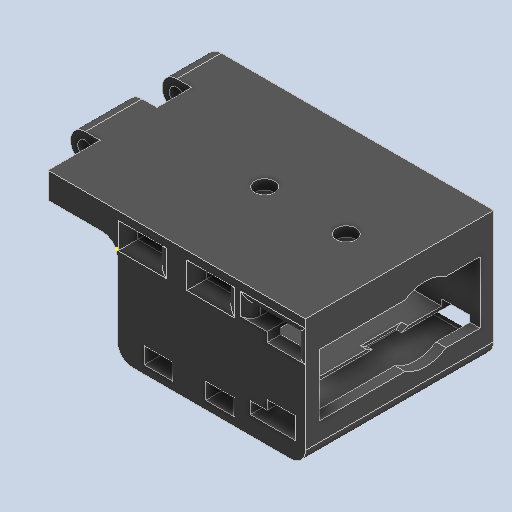
# Autodesk Inventor part: Base - version 2
Saved by Autodesk Inventor 2026 (Build 300175050, 175E)
## iProperties
Created: 2025-10-13
Part Number: Base - version 2
Material: Plastico PETG
Document SubType Name: Modeling
Designer: bello
Density: 1.27 g/cm^3
Appearance: Genérico
Author: bello
Autodesk Inventor part; units mm, degrees
ref_plane "YZ Plane" through (0, 0, 0) normal (1, 0, 0) x (0, 1, 0)
sketch "Boceto1" plane through (0, 0, 0) normal (0, 1, 0) x (-1, 0, 0)
  line L0 (0, 0) -> (-38, 0)
  line L1 (-38, 0) -> (-38, -38)
  line L2 (-38, -38) -> (0, -38)
  line L3 (0, -38) -> (0, 0)
  dimension "d0" = 38
  dimension "d1" = 38
  constraints: 8 end point, 2 parallel, 1 horizontal, 1 perpendicular
  measures "d0" distance of L2.end L0.start
  measures "d1" distance of L0.start L0.end
extrude "Extrusión1" add sketch "Boceto1" along normal blind 26
sketch "Boceto2" plane through (38, 0, 0) normal (1, 0, 0) x (0, 0, -1)
  line L0 (7.25, 19.25) -> (30.75, 19.25)
  line L1 (30.75, 19.25) -> (30.75, 6.75)
  line L2 (30.75, 6.75) -> (7.25, 6.75)
  line L3 (7.25, 6.75) -> (7.25, 19.25)
  line L4 (0, 26) -> (38, 26) projected
  line L5 (19, 26) -> (19, 0)
  line L6 (0, 0) -> (38, 0) projected
  line L7 (0, 0) -> (0, 26) projected
  line L8 (0, 13) -> (38, 13)
  line L9 (38, 0) -> (38, 26) projected
  dimension "d4" = 23.5
  dimension "d5" = 12.5
  dimension "d6" = 23.5
  dimension "d7" = 12.5
  constraints: 12 end point, 4 midpoint, 2 parallel, 1 horizontal, 1 perpendicular
  measures "d4" distance of L0.start L0.end
  measures "d5" distance of L2.end L0.start
  measures "d6" diameter of L3 L5
  measures "d7" diameter of L2 L8
extrude "Extrusión2" cut sketch "Boceto2" against normal blind 36.5 contours L0 L5 L8 L3 | L0 L1 L8 L5 | L8 L5 L2 L3 | L8 L1 L2 L5
sketch "Boceto3" plane through (38, 0, 0) normal (1, 0, 0) x (0, 0, -1)
  line L0 (7.25, 19.25) -> (30.75, 19.25) projected
  line L1 (19, 19.25) -> (19, 6.75)
  line L2 (30.75, 6.75) -> (7.25, 6.75) projected
  line L3 (2.75, 6.75) -> (35.25, 6.75)
  line L4 (35.25, 6.75) -> (35.25, 19.25)
  line L5 (35.25, 19.25) -> (2.75, 19.25)
  line L6 (2.75, 19.25) -> (2.75, 6.75)
  line L7 (2.75, 6.75) -> (35.25, 19.25) construction
  line L8 (35.25, 6.75) -> (2.75, 19.25) construction
  point P0 (0, 0)
  point P1 (19, 13)
  point P2 (7.25, 6.75)
  point P3 (7.25, 19.25)
  dimension "d10" = 32.5
  constraints: 14 end point, 5 midpoint, 2 parallel, 1 horizontal, 1 perpendicular
  measures "d10" distance of L5.end L4.end
extrude "Extrusión3" cut sketch "Boceto3" against normal blind 19
sketch "Boceto5" plane through (19, 0, 0) normal (1, 0, 0) x (0, 0, -1)
  line L0 (2.75, 6.75) -> (2.75, 19.25) projected
  line L1 (2.75, 13) -> (35.25, 13)
  line L2 (35.25, 19.25) -> (35.25, 6.75) projected
  line L3 (7.25, 19.25) -> (7.25, 6.75) projected
  circle A0 centre (5.35, 13) radius 0.8
  circle A1 centre (32.65, 13) radius 0.8
  point P0 (0, 0)
  dimension "d16" = 4.5
  dimension "d17" = 1.6
  dimension "d18" = 2.6
  dimension "d19" = 2.6
  dimension "d20" = 1.6
  constraints: 2 centre point, 2 end point, 2 midpoint, 2 point on line
  measures "d16" distance between parallel lines of L3 L0
  measures "d17" diameter of A0
  measures "d18" distance from line of L0 A0.centre
  measures "d19" distance from line of L2 A1.centre
  measures "d20" diameter of A1
extrude "Extrusión5" cut sketch "Boceto5" against normal blind 5.7
sketch "Boceto6" plane through (38, 0, 0) normal (1, 0, 0) x (0, 0, -1)
  line L0 (0, 0) -> (0, 26) projected
  line L1 (0, 13) -> (38, 13)
  line L2 (38, 0) -> (38, 26) projected
  circle A0 centre (24.25, 13) radius 7.5
  line L3 (2.75, 6.75) -> (2.75, 19.25) projected
  line L4 (35.25, 19.25) -> (35.25, 6.75) projected
  dimension "d24" = 15
  dimension "d30" = 11
  constraints: 2 end point, 2 midpoint, 1 centre point, 1 point on line
  measures "d24" diameter of A0
  measures "d30" distance from line of L4 A0.centre
extrude "Extrusión6" cut sketch "Boceto6" against normal blind 9
sketch "Boceto9" plane through (38, 0, 0) normal (1, 0, 0) x (0, 0, -1)
  line L0 (28.9453, 7.1) -> (48.9575, 7.1)
  arc A0 (28.3958, 19.25) -> (20.1042, 19.25) centre (24.25, 13) ccw projected
  circle A1 centre (24.25, 13) radius 3.7369
  line L1 (29.3531, 3.4386) -> (49.9663, 3.4386)
  point P0 (0, 0)
  dimension "d31" = 5.9
  dimension "d32" = 3.6614
  dimension "d33" = 9.0792
  constraints: 4 end point, 2 horizontal, 1 centre point, 1 coincident
  measures "d31" distance from line of L0 A1.centre
  measures "d32" distance between parallel lines of L1 L0
sketch "Boceto12" plane through (38, 0, -38) normal (0, 0, -1) x (-1, 0, 0)
  line L0 (31.8255, 18) -> (36.5, 18)
  line L1 (36.5, 18) -> (36.5, 8)
  line L2 (36.5, 8) -> (31.8255, 8)
  line L3 (31.8255, 8) -> (31.8255, 18)
  line L4 (38, 0) -> (38, 26) projected
  line L5 (38, 13) -> (26.3791, 13)
  dimension "d52" = 1.5
  dimension "d57" = 5
  dimension "d58" = 10
  constraints: 10 end point, 2 horizontal, 2 parallel, 1 midpoint, 1 perpendicular
  measures "d52" distance between parallel lines of L1 L4
  measures "d57" distance between parallel lines of L5 L0
  measures "d58" distance of L2.end L0.start
extrude "Extrusión10" cut sketch "Boceto12" against normal blind 10
sketch "Boceto10" plane through (38, 0, -38) normal (0, 0, -1) x (-1, 0, 0)
  line L0 (2.05, 8) -> (7.75, 8)
  line L1 (7.75, 8) -> (7.75, 3.7)
  line L2 (7.75, 3.7) -> (2.05, 3.7)
  line L3 (2.05, 3.7) -> (2.05, 8)
  line L4 (0, 0) -> (0, 26) projected
  line L5 (38, 0) -> (38, 26) projected
  line L6 (0, 0) -> (38, 0) projected
  line L7 (14.45, 1.7) -> (20.15, 1.7)
  line L8 (20.15, 1.7) -> (20.15, 5)
  line L9 (20.15, 5) -> (14.45, 5)
  line L10 (14.45, 5) -> (14.45, 1.7)
  line L11 (26.85, 1.7) -> (32.55, 1.7)
  line L12 (32.55, 1.7) -> (32.55, 5)
  line L13 (32.55, 5) -> (26.85, 5)
  line L14 (26.85, 5) -> (26.85, 1.7)
  line L15 (38, 13) -> (0, 13)
  line L16 (7.75, 3.7) -> (11.15, 3.7)
  line L17 (11.15, 3.7) -> (11.15, 6.1)
  line L18 (11.15, 6.1) -> (7.75, 6.1)
  line L19 (7.75, 6.1) -> (7.75, 3.7)
  line L20 (2.05, 8) -> (7.75, 3.7)
  line L21 (7.75, 8) -> (2.05, 3.7)
  line L22 (14.45, 5) -> (20.15, 1.7)
  line L23 (14.45, 1.7) -> (20.15, 5)
  line L24 (26.85, 5) -> (32.55, 1.7)
  line L25 (26.85, 1.7) -> (32.55, 5)
  point P0 (29.7, 3.35)
  point P1 (17.3, 3.35)
  point P2 (4.9, 5.85)
  dimension "d35" = 4.3
  dimension "d36" = 5.7
  dimension "d39" = 2.05
  dimension "d49" = 3.3
  dimension "d59" = 5
  dimension "d61" = 3.7
  dimension "d62" = 1.7
  dimension "d63" = 6.7
  dimension "d64" = 6.7
  dimension "d65" = 5.7
  dimension "d66" = 5.7
  dimension "d67" = 3.3
  dimension "d134" = 3.4
  dimension "d135" = 2.4
  dimension "d148" = 8.3
  dimension "d149" = 20.7
  dimension "d150" = 4.9
  constraints: 46 end point, 8 parallel, 5 midpoint, 4 horizontal, 4 perpendicular, 2 point on line
  measures "d35" distance between parallel lines of L0 L2
  measures "d36" distance of L0.start L0.end
  measures "d39" distance between parallel lines of L4 L3
  measures "d49" distance of L9.end L7.start
  measures "d59" distance between parallel lines of L15 L0
  measures "d61" distance between parallel lines of L6 L2
  measures "d62" distance between parallel lines of L6 L7
  measures "d63" distance between parallel lines of L1 L10
  measures "d64" distance between parallel lines of L8 L14
  measures "d65" distance of L8.end L9.end
  measures "d66" distance of L12.end L13.end
  measures "d67" distance of L11.end L12.end
  measures "d134" distance of L18.end L17.end
  measures "d135" distance of L16.end L17.end
  measures "d148" distance from line of L5 point (29.7, 3.35)
  measures "d149" distance from line of L5 point (17.3, 3.35)
  measures "d150" distance from line of L4 point (4.9, 5.85)
extrude "Extrusión8" cut sketch "Boceto10" against normal through all contours L20 L21 L3 | L0 L21 L20 | L1 L20 L21 | L21 L20 L2 | L18 L17 L16 L1 | L23 L22 L7 | L10 L22 L23 | L22 L23 L8 | L9 L23 L22 | L25 L24 L11 | L14 L24 L25 | L24 L25 L12 | L13 L25 L24
sketch "Boceto11" plane through (0, 0, 0) normal (0, 0, 1) x (1, 0, 0)
  line L0 (0, 0) -> (0, 26) projected
  line L1 (38, 0) -> (38, 26) projected
  line L2 (30.25, 22.3) -> (35.95, 22.3)
  line L3 (35.95, 22.3) -> (35.95, 18)
  line L4 (35.95, 18) -> (30.25, 18)
  line L5 (30.25, 18) -> (30.25, 22.3)
  line L6 (21.75, 24.3) -> (16.05, 24.3)
  line L7 (16.05, 24.3) -> (16.05, 21)
  line L8 (16.05, 21) -> (21.75, 21)
  line L9 (21.75, 21) -> (21.75, 24.3)
  line L10 (7.85, 24.3) -> (2.15, 24.3)
  line L11 (2.15, 24.3) -> (2.15, 21)
  line L12 (2.15, 21) -> (7.85, 21)
  line L13 (7.85, 21) -> (7.85, 24.3)
  line L14 (0, 26) -> (38, 26) projected
  line L15 (30.25, 22.3) -> (26.85, 22.3)
  line L16 (26.85, 22.3) -> (26.85, 19.9)
  line L17 (26.85, 19.9) -> (30.25, 19.9)
  line L18 (30.25, 19.9) -> (30.25, 22.3)
  line L19 (2.15, 24.3) -> (7.85, 21)
  line L20 (7.85, 24.3) -> (2.15, 21)
  line L21 (16.05, 24.3) -> (21.75, 21)
  line L22 (21.75, 24.3) -> (16.05, 21)
  line L23 (30.25, 22.3) -> (35.95, 18)
  line L24 (30.25, 18) -> (35.95, 22.3)
  point P0 (0, 13)
  point P1 (33.1, 20.15)
  point P2 (5, 22.65)
  point P3 (18.9, 22.65)
  dimension "d42" = 4.3
  dimension "d43" = 5.7
  dimension "d45" = 2.05
  dimension "d60" = 5
  dimension "d68" = 8.2
  dimension "d69" = 8.5
  dimension "d70" = 5.7
  dimension "d71" = 5.7
  dimension "d72" = 3.3
  dimension "d73" = 1.7
  dimension "d131" = 2
  dimension "d132" = 3.4
  dimension "d133" = 2.4
  dimension "d151" = 4.9
  dimension "d152" = 5
  dimension "d153" = 18.9
  constraints: 44 end point, 9 parallel, 4 horizontal, 4 midpoint, 4 perpendicular, 3 point on line
  measures "d42" distance of L4.end L2.start
  measures "d43" distance of L2.start L2.end
  measures "d45" distance between parallel lines of L1 L3
  measures "d60" distance from line of point (0, 13) L4
  measures "d68" distance between parallel lines of L13 L7
  measures "d69" distance between parallel lines of L5 L9
  measures "d70" distance of L7.end L8.end
  measures "d71" distance of L11.end L12.end
  measures "d72" distance of L10.end L11.end
  measures "d73" distance between parallel lines of L10 L14
  measures "d131" distance between parallel lines of L2 L6
  measures "d132" distance of L2.start L15.end
  measures "d133" distance of L15.end L16.end
  measures "d151" distance from line of L1 point (33.1, 20.15)
  measures "d152" distance from line of L0 point (5, 22.65)
  measures "d153" distance from line of L0 point (18.9, 22.65)
extrude "Extrusión9" cut sketch "Boceto11" against normal through all
sketch "Boceto15" plane through (0, 26, 0) normal (0, 1, 0) x (1, 0, 0)
  line L0 (0, 0) -> (38, 0) projected
  line L1 (19, 0) -> (19, 38)
  line L2 (38, 38) -> (0, 38) projected
  circle A0 centre (19, 19) radius 8.25
  circle A1 centre (27.25, 19) radius 2
  circle A2 centre (10.75, 19) radius 2
  circle A3 centre (19, 10.75) radius 2
  circle A4 centre (19, 27.25) radius 2
  dimension "d81" = 16.5
  dimension "d82" = 4
  dimension "d83" = 4
  dimension "d84" = 4
  dimension "d85" = 4
  constraints: 5 centre point, 4 point on circle, 3 midpoint, 2 end point, 2 point on line
  measures "d81" diameter of A0
  measures "d82" diameter of A1
  measures "d83" diameter of A2
  measures "d84" diameter of A3
  measures "d85" diameter of A4
extrude "Extrusión13" cut sketch "Boceto15" against normal blind 2 contours A2 A0 | A0 A2 | A1 A0 | A0 A1
sketch "Boceto22" plane through (38, 0, -38) normal (0, 0, -1) x (-1, 0, 0)
  line L0 (38, 26) -> (55, 26)
  arc A0 (55, 20) -> (55, 26) centre (55, 23) ccw
  circle A1 centre (55, 23) radius 3
  line L1 (38, 0) -> (38, 26) projected
  line L2 (38, 20.731) -> (53.0374, 20.731)
  circle A2 centre (55, 23) radius 1.5
  point P0 (55, 20)
  dimension "d103" = 17
  dimension "d104" = 6
  dimension "d105" = 3
  dimension "d106" = 5.269
  dimension "d107" = 3
  constraints: 4 end point, 2 centre point, 2 coincident, 2 horizontal, 2 point on circle, 1 point on line, 5 other
  measures "d103" distance of L0.start L0.end
  measures "d104" distance of L0.end A0.start
  measures "d105" radius of A0
  measures "d106" distance between parallel lines of L2 L0
  measures "d107" diameter of A2
extrude "Extrusión19" add sketch "Boceto22" against normal blind 38
ref_plane "Plano de trabajo4" through (38, 0, -22) normal (0, 0, -1) x (-1, 0, 0)
sketch "Boceto25" plane through (38, 0, -22) normal (0, 0, -1) x (-1, 0, 0)
  arc A0 (53.0374, 20.731) -> (55, 26) centre (55, 23) ccw projected
  circle A1 centre (55, 23) radius 3
  line L0 (53.0374, 20.731) -> (38, 20.731) projected
  line L1 (53.0374, 20.731) -> (52, 20.731)
  line L2 (52, 20.731) -> (52, 26)
  line L3 (0, 26) -> (55, 26) projected
  line L4 (52, 26) -> (55, 26)
  point P0 (38, 0)
  constraints: 6 end point, 2 perpendicular, 2 point on line, 1 centre point, 1 coincident, 1 tangent
extrude "Extrusión22" cut sketch "Boceto25" along normal blind 7
sketch "Boceto26" plane through (0, 0, 0) normal (0, 0, 1) x (1, 0, 0)
  circle A0 centre (-17, 23) radius 1.5 projected
  line L0 (38, 26) -> (-17, 26) projected
  circle A1 centre (-17, 23) radius 3
  line L1 (0, 20.731) -> (-15.0374, 20.731) projected
  line L2 (-15.0374, 20.731) -> (-14, 20.731)
  line L3 (-14, 20.731) -> (-14, 26)
  line L4 (-14, 26) -> (-17, 26)
  point P0 (0, 0)
  constraints: 6 end point, 2 perpendicular, 2 point on line, 1 centre point, 1 coincident, 1 point on circle, 1 tangent
extrude "Extrusión23" cut sketch "Boceto26" against normal blind 10.5
ref_plane "Plano de trabajo5" through (38, 0, -19) normal (0, 0, -1) x (-1, 0, 0)
sketch "Boceto27" plane through (38, 0, -19) normal (0, 0, -1) x (-1, 0, 0)
  circle A0 centre (55, 23) radius 1.5 projected
  line L0 (38, 20.731) -> (43.7201, 20.731)
  line L1 (55, 20.731) -> (44.323, 20.731)
  line L2 (38, 20.731) -> (53.0374, 20.731) projected
  line L3 (44.323, 20.731) -> (39.1014, 5.5749)
  line L4 (39.1014, 5.5749) -> (38, 5.5749)
  line L5 (38, 0) -> (38, 20.731) projected
  line L6 (38, 5.5749) -> (38, 20.731)
  line L7 (38, 20.731) -> (44.323, 20.731)
  dimension "d125" = 10.677
  dimension "d126" = 16.0304
  dimension "d127" = 109.01
  constraints: 12 end point, 2 point on line, 1 collinear, 1 horizontal, 1 parallel, 1 perpendicular, 1 other
  measures "d125" distance of L1.start L1.end
  measures "d126" distance of L1.end L3.end
  measures "d127" angle of L3 L4
extrude "Extrusión24" add sketch "Boceto27" along normal mid plane 15 contours L0 L2 L3 L4 L5
sketch "Boceto28" plane through (38, 19.25, -20.1042) normal (0, -1, 0) x (1, 0, 0)
  point P0 (-38, 20.1042)
fillet "Empalme4" radius 2 3 edges at (35.95, 20.15, 0) (31.4, 22.3, 0) (26.85, 21.1, 0)
fillet "Empalme5" radius 1.8 8 edges at (20.7, 5, -38) (23.55, 3.35, -38) (20.7, 1.7, -38) (17.85, 3.35, -38) (11.15, 3.35, -38) (8.3, 5, -38) (5.45, 3.35, -38) (8.3, 1.7, -38)
fillet "Empalme7" radius 2 6 edges at (2.15, 22.65, 0) (5, 21, 0) (7.85, 22.65, 0) (16.05, 22.65, 0) (18.9, 21, 0) (21.75, 22.65, 0)
fillet "Empalme8" radius 3 2 edges at (0, 20.731, -32.25) (0, 20.731, -5.75)
fillet "Empalme9" radius 3 2 edges at (0, 0, -19) (38, 0, -19)
sketch "Boceto31" plane through (38, 0, -26.5) normal (0, 0, -1) x (-1, 0, 0)
  line L0 (39.1014, 5.5749) -> (38, 5.5749) projected
  line L1 (39.1014, 5.5749) -> (39.6306, 21.662) construction
  line L2 (44.323, 20.731) -> (41, 20.731) projected
  line L3 (39.6306, 21.662) -> (44.323, 20.731) construction
  spline S0 degree 2 poles (39.1014, 5.5749) (39.6306, 21.662) (44.323, 20.731) knots 1 1 1 2 2 2
  line L4 (44.323, 20.731) -> (39.1014, 5.5749)
  line L5 (44.323, 20.731) -> (41.4441, 20.731)
  point P0 (38, 0)
  point P1 (43.346, 20.731)
  constraints: 4 end point, 1 point on line, 3 other
extrude "Extrusión27" cut sketch "Boceto31" against normal through all contours L4 S0 L2
fillet "Empalme10" radius 2 2 edges at (35.95, 5.85, -38) (31.4, 3.7, -38)
fillet "Empalme11" radius 1.5 1 edges at (26.85, 3.9, -38)
